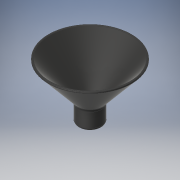
# Autodesk Inventor part: entonnoir
Saved by Autodesk Inventor 2019 (Build 230136000, 136)
## iProperties
Created: 2021-01-18
Part Number: entonnoir
Material: Générique
Document SubType Name: Modeling
Designer: tristan.cremona
Density: 1 g/cm^3
Appearance: Lisse - Noir
Author: tristan.cremona
Autodesk Inventor part; units mm, degrees
ref_plane "YZ Plane" through (0, 0, 0) normal (1, 0, 0) x (0, 1, 0)
ref_plane "XZ Plane" through (0, 0, 0) normal (0, 1, 0) x (-1, 0, 0)
ref_plane "XY Plane" through (0, 0, 0) normal (0, 0, 1) x (1, 0, 0)
sketch "Esquisse2" plane through (0, 0, 0) normal (1, 0, 0) x (0, 1, 0)
  line L0 (0, -10) -> (17, -10)
  line L1 (17, -7) -> (62.9627, -45.5673)
  line L2 (17, -7) -> (77, -7) construction
  line L3 (62.9627, -45.5673) -> (61.4855, -47.3277)
  line L4 (61.4855, -47.3277) -> (17, -10)
  line L5 (17, -10) -> (17, -13)
  line L6 (17, -13) -> (20.5753, -13)
  line L7 (17, -13) -> (0, -13)
  line L8 (0, -13) -> (0, -10)
  line L9 (17, -7) -> (17, -10)
  line L10 (0, 0) -> (24.971, 0)
  dimension "d0" = 10
  dimension "d1" = 17
  dimension "d2" = 40
  dimension "d4" = 3
  dimension "d5" = 60
  dimension "d7" = 3
  dimension "d8" = 7
  constraints: 22 end point, 3 horizontal, 3 perpendicular, 2 point on line, 2 vertical, 1 equal length, 1 parallel
  measures "d0" distance of L10.start L0.start
  measures "d1" distance of L0.start L0.end
  measures "d2" angle of L1 L2
  measures "d4" distance of L0.end L5.end
  measures "d5" distance of L1.start L1.end
  measures "d7" distance of L1.start L0.end
  measures "d8" distance from line of L10 L1.start
revolve "Révolution1" add sketch "Esquisse2" angle 360 about axis through (0, 0, 0) along (0, 1, 0)
fillet "Congé1" radius 5 1 edges at (0, 20.5753, 13)
fillet "Congé2" radius 3 1 edges at (0, 0, 13)
fillet "Congé3" radius 1.1 2 edges at (0, 61.4855, 47.3277) (0, 62.9627, 45.5673)
